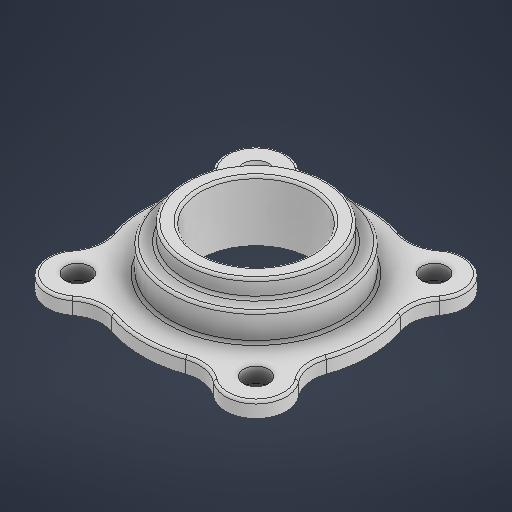
# Autodesk Inventor part: DP806
Saved by Autodesk Inventor 2025.4 (Build 294407000, 407)
## iProperties
Created: 2026-05-07
Part Number: DP806
Material: Generic
Document SubType Name: Modeling
Designer: VuQuan
Density: 1 g/cm^3
Appearance: Default
Author: VuQuan
Autodesk Inventor part; units mm, degrees
ref_plane "YZ Plane" through (0, 0, 0) normal (1, 0, 0) x (0, 1, 0)
ref_plane "XZ Plane" through (0, 0, 0) normal (0, 1, 0) x (-1, 0, 0)
ref_plane "XY Plane" through (0, 0, 0) normal (0, 0, 1) x (1, 0, 0)
sketch "Sketch1" plane through (0, 0, 0) normal (0, 0, 1) x (1, 0, 0)
  line L0 (0, 0) -> (0, 12) construction
  line L1 (11, 3) -> (11, 12)
  line L2 (11, 12) -> (14, 12)
  line L3 (14, 12) -> (14, 8.5)
  line L4 (14, 8.5) -> (17, 8.5)
  line L5 (17, 8.5) -> (17, 3)
  line L6 (11, 3) -> (17, 3)
  dimension "d0" = 22
  dimension "d1" = 28
  dimension "d2" = 3.5
  dimension "d3" = 34
  dimension "d4" = 5.5
  dimension "d5" = 3
  constraints: 14 end point, 2 perpendicular, 2 vertical, 1 horizontal, 1 point on line
  measures "d0" diameter of L1 L0
  measures "d1" diameter of L3 L0
  measures "d2" distance between parallel lines of L2 L4
  measures "d3" diameter of L5 L0
  measures "d4" distance of L4.end L5.end
  measures "d5" distance from line of L0.start L6
revolve "Revolution1" add sketch "Sketch1" angle 360 about axis through (0, 0, 0) along (0, 1, 0)
sketch "Sketch2" plane through (0, 3, 0) normal (0, -1, 0) x (1, 0, 0)
  circle A0 centre (0, 0) radius 17 projected
  circle A1 centre (0, 0) radius 11 projected
  circle A2 centre (17.6777, 17.6777) radius 2.5
  arc A3 (22.3887, 13.962) -> (13.962, 22.3887) centre (17.6777, 17.6777) ccw
  arc A4 (21.2682, -7.3427) -> (21.2682, 7.3427) centre (0, 0) ccw
  arc A5 (22.3887, 13.962) -> (21.2682, 7.3427) centre (27.8849, 9.6271) ccw
  arc A6 (7.3427, 21.2682) -> (13.962, 22.3887) centre (9.6271, 27.8849) ccw
  circle A7 centre (-17.6777, 17.6777) radius 2.5
  arc A8 (-13.962, 22.3887) -> (-22.3887, 13.962) centre (-17.6777, 17.6777) ccw
  arc A9 (7.3427, 21.2682) -> (-7.3427, 21.2682) centre (0, 0) ccw
  arc A10 (-13.962, 22.3887) -> (-7.3427, 21.2682) centre (-9.6271, 27.8849) ccw
  arc A11 (-21.2682, 7.3427) -> (-22.3887, 13.962) centre (-27.8849, 9.6271) ccw
  circle A12 centre (-17.6777, -17.6777) radius 2.5
  arc A13 (-22.3887, -13.962) -> (-13.962, -22.3887) centre (-17.6777, -17.6777) ccw
  arc A14 (-21.2682, 7.3427) -> (-21.2682, -7.3427) centre (0, 0) ccw
  arc A15 (-22.3887, -13.962) -> (-21.2682, -7.3427) centre (-27.8849, -9.6271) ccw
  arc A16 (-7.3427, -21.2682) -> (-13.962, -22.3887) centre (-9.6271, -27.8849) ccw
  circle A17 centre (17.6777, -17.6777) radius 2.5
  arc A18 (13.962, -22.3887) -> (22.3887, -13.962) centre (17.6777, -17.6777) ccw
  arc A19 (-7.3427, -21.2682) -> (7.3427, -21.2682) centre (0, 0) ccw
  arc A20 (13.962, -22.3887) -> (7.3427, -21.2682) centre (9.6271, -27.8849) ccw
  arc A21 (21.2682, -7.3427) -> (22.3887, -13.962) centre (27.8849, -9.6271) ccw
  circle A22 centre (0, 0) radius 25 construction
  point P0 (21.2682, -7.3427)
  point P1 (-7.3427, -21.2682)
  dimension "d7" = 5
  dimension "d8" = 6
  dimension "d9" = 7
  dimension "d10" = 22.5
  dimension "d13" = 360
  constraints: 32 point on circle, 20 centre point, 7 coincident, 5 tangent, 1 equal radius, 1 vertical alignment, 64 other
  measures "d7" diameter of A2
  measures "d8" radius of A3
  measures "d9" radius of A5
  measures "d10" radius of A4
extrude "Extrusion1" add sketch "Sketch2" along normal blind 3 contours A0 | A5 A4 A21 A18 A20 A19 A16 A13 A15 A14 A11 A8 A10 A9 A6 A3
fillet "Fillet1" radius 0.5 21 edges at (-10.7955, 3, 20.9831) (-21.9203, 3, 21.9203) (-20.9831, 3, 10.7955) (-22.5, 3, 0) (-20.9831, 3, -10.7955) (-21.9203, 3, -21.9203) (-10.7955, 3, -20.9831) (0, 3, -22.5) (10.7955, 3, -20.9831) (21.9203, 3, -21.9203) (20.9831, 3, -10.7955) (22.5, 3, 0) (20.9831, 3, 10.7955) (21.9203, 3, 21.9203) (10.7955, 3, 20.9831) (0, 3, 22.5) (-17, 8.5, 0) (-14, 12, 0) (-11, 12, 0) (-17, 3, 0) (-14, 8.5, 0)
body "Solid1"
